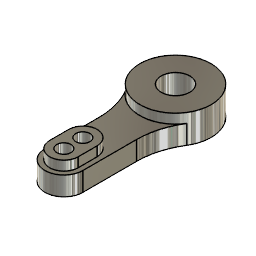
サーボハンドル (Autodesk Fusion 360 design; units mm, degrees)
Autodesk Fusion 360 part; units mm, degrees
sketch "スケッチ1" plane through (0, 0, 0) normal (0, 0, 1) x (1, 0, 0)
  line L0 (0, 0) -> (15, 0)
  line L1 (15, 0) -> (15, 35)
  line L2 (15, 35) -> (0, 35)
  line L3 (0, 35) -> (0, 0)
  circle A0 centre (7.5, 27.5) radius 7.5
  line L4 (3.5, 0) -> (11.5, 0)
  line L5 (11.5, 0) -> (11.5, 21.1557)
  line L6 (11.5, 21.1557) -> (3.5, 21.1557)
  line L7 (3.5, 21.1557) -> (3.5, 0)
  dimension "d1" = 8
  dimension "d2" = 3.5
  dimension "d4" = 35
  dimension "d5" = 15
  constraint horizontal L0
  constraint vertical L1
  constraint horizontal L2
  constraint vertical L3
  constraint coincident L0.start L3.end
  constraint tangent L3 A0
  constraint tangent L2 A0
  constraint horizontal L4
  constraint vertical L5
  constraint horizontal L6
  constraint vertical L7
  constraint coincident L0 L4.start
  constraint coincident A0 L6.end
  measures "d1" distance of L5.end L6.end
  measures "d2" distance of L3 L7
  measures "d4" distance of L2 L4
  measures "d5" diameter of A0
extrude "押し出し1" add sketch "スケッチ1" along normal blind 6 contours L0 A0 L4 L5 L7 | A0 L6 | A0 L6
fillet "フィレット1" radius 15.5 2 edges at (3.5, 21.1557, 3) (11.5, 21.1557, 3)
fillet "フィレット1" radius 4 2 edges at (3.5, 0, 3) (11.5, 0, 3)
sketch "スケッチ2" plane through (0, 0, 6) normal (0, 0, 1) x (-1, 0, 0)
  arc A0 (-3.5, -4) -> (-11.5, -4) centre (-7.5, -4) ccw
  line L0 (-11.5, -4) -> (-11.5, -15.3037)
  arc A1 (-13.8587, -23.5229) -> (-11.5, -15.3037) centre (-27, -15.3037) ccw
  arc A2 (-13.8587, -23.5229) -> (-1.1413, -23.5229) centre (-7.5, -27.5) ccw
  arc A3 (-3.5, -15.3037) -> (-1.1413, -23.5229) centre (12, -15.3037) ccw
  line L1 (-3.5, -15.3037) -> (-3.5, -4)
  line L2 (-10.5, -4) -> (-10.5, -8)
  line L3 (-4.5, -8) -> (-4.5, -4)
  arc A4 (-4.5, -4) -> (-7.5, -1) centre (-7.5, -4) ccw
  arc A5 (-7.5, -1) -> (-10.5, -4) centre (-7.5, -4) ccw
  arc A6 (-7.5, -11) -> (-4.5, -8) centre (-7.5, -8) ccw
  arc A7 (-10.5, -8) -> (-7.5, -11) centre (-7.5, -8) ccw
  circle A8 centre (-7.5, -27.5) radius 7.5
  point P0 (-4.5, -1)
  point P1 (-10.5, -1)
  point P2 (-4.5, -11)
  dimension "d12" = 6
  dimension "d13" = 10
  dimension "d14" = 1
  dimension "d16" = 3
  constraint vertical L2
  constraint vertical L3
  constraint coincident P0 L3
  constraint tangent L3 A4
  constraint coincident P1 L2
  constraint tangent L2 A5
  constraint equal A4 A5
  constraint coincident A4.end A5.start
  constraint coincident P2 L3
  constraint tangent L3 A6
  constraint equal A4 A6
  constraint tangent L2 A7
  constraint equal A4 A7
  constraint coincident A6.start A7.end
  measures "d12" distance of P0 P1
  measures "d13" distance of P0 P2
  measures "d14" distance of L1 L3
  measures "d16" radius of A4
extrude "押し出し2" cut sketch "スケッチ2" against normal blind 2 contours A0 L0 A1 A3 L1 A8
sketch "スケッチ3" plane through (0, 0, 6) normal (0, 0, 1) x (-1, 0, 0)
  line L0 (-10.5, -4) -> (-10.5, -8)
  arc A0 (-10.5, -8) -> (-4.5, -8) centre (-7.5, -8) ccw
  line L1 (-4.5, -8) -> (-4.5, -4)
  arc A1 (-4.5, -4) -> (-10.5, -4) centre (-7.5, -4) ccw
  circle A2 centre (-7.5, -8) radius 1.5
  circle A3 centre (-7.5, -4) radius 1.5
  line L2 (-7.5, -8) -> (-7.5, -4)
  line L3 (-4, 0) -> (-13, 0)
  arc A4 (-3.5, -4) -> (-11.5, -4) centre (-7.5, -4) ccw
  circle A5 centre (-7.5, -27.5) radius 3
  circle A6 centre (-7.5, -27.5) radius 7.5
  dimension "d20" = 4
  dimension "d21" = 3
  dimension "d22" = 3
  dimension "d23" = 3
  dimension "d24" = 4
  dimension "d27" = 6
  constraint coincident A0.centre A2.centre
  constraint coincident A1.centre A3.centre
  constraint parallel L1 L2
  constraint horizontal L3
  constraint tangent L3 A4
  constraint concentric A5 A6
  measures "d20" distance of A0.centre A1.centre
  measures "d21" diameter of A2
  measures "d22" diameter of A3
  measures "d23" distance of L1 L2
  measures "d24" distance of A1.centre L3
  measures "d27" diameter of A5
extrude "押し出し3" cut sketch "スケッチ3" against normal blind 6 contours A2 | A3 | A5
